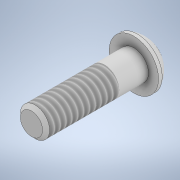
# Autodesk Inventor part: DERKS Axle Peg
Saved by Autodesk Inventor 2020 (Build 240168000, 168)
## iProperties
Created: 2020-04-30
Part Number: DERKS Axle Peg
Material: Generic
Document SubType Name: Modeling
Designer: tader
Density: 1 g/cm^3
Appearance: Default
Author: tader
Autodesk Inventor part; units mm, degrees
ref_plane "YZ Plane" through (0, 0, 0) normal (1, 0, 0) x (0, 1, 0)
ref_plane "XZ Plane" through (0, 0, 0) normal (0, 1, 0) x (-1, 0, 0)
ref_plane "XY Plane" through (0, 0, 0) normal (0, 0, 1) x (1, 0, 0)
sketch "Sketch1" plane through (0, 0, 0) normal (0, 1, 0) x (-1, 0, 0)
  line L0 (-1.3816, -12.6421) -> (1.7934, -12.6421)
  line L1 (1.7934, -12.6421) -> (1.7934, 12.7579)
  line L2 (1.7934, 12.7579) -> (-1.3816, 12.7579)
  line L3 (-1.3816, 12.7579) -> (-1.3816, -9.4671)
  line L4 (-1.3816, -9.4671) -> (-3.566, -9.4671)
  line L5 (-3.566, -9.4671) -> (-3.566, -10.2545)
  arc A0 (-3.566, -10.2545) -> (-1.3816, -12.6421) centre (1.7847, -7.5522) ccw
  point P0 (0, 0)
  dimension "d0" = 25.4
  dimension "d1" = 5.3594
  dimension "d2" = 0.7874
  dimension "d3" = 3.175
  dimension "d4" = 3.175
  dimension "d5" = 5.9944
  dimension "d6" = 3.175
  constraints: 12 end point, 5 perpendicular, 2 point on circle, 1 centre point, 1 horizontal
  measures "d0" distance of L0.end L1.end
  measures "d1" distance between parallel lines of L1 L5
  measures "d2" distance of L4.end L5.end
  measures "d3" distance of L0.start L0.end
  measures "d4" distance between parallel lines of L1 L3
  measures "d5" radius of A0
  measures "d6" vertical distance of L4.end L0.start
revolve "Revolution1" add sketch "Sketch1" angle 360 about axis through (-1.7934, 0, -12.6421) along (0, 0, 1)
sketch "Sketch2" plane through (-1.7934, 0, -12.6421) normal (0, 0, -1) x (-1, 0, 0)
  line L0 (-0.018, 2.2876) -> (1.9721, 1.1594)
  line L1 (1.9721, 1.1594) -> (1.9902, -1.1282)
  line L2 (1.9902, -1.1282) -> (0.018, -2.2876)
  line L3 (0.018, -2.2876) -> (-1.9721, -1.1594)
  line L4 (-1.9721, -1.1594) -> (-1.9902, 1.1282)
  line L5 (-1.9902, 1.1282) -> (-0.018, 2.2876)
  point P0 (-1.7934, 0)
  point P1 (0, 0)
  dimension "d8" = 3.9624
  constraints: 12 end point, 13 other
  measures "d8" distance between parallel lines of L2 L5
extrude "Extrusion1" cut sketch "Sketch2" against normal blind 2.8194
chamfer "Chamfer1" distance 0.762 angle 45 1 edges at (-4.9684, 0, 12.7579)
thread "Thread1" size "1/4-20 UNC" class "2A" standard "ANSI Unified Screw Threads" length 25.4 offset 6.35
body "Solid1"
